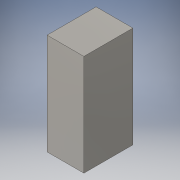
# Autodesk Inventor part: Motor
Saved by Autodesk Inventor 2016 (Build 200138000, 138)
## iProperties
Created: 2016-08-06
Part Number: Motor
Material: Stainless Steel
Document SubType Name: Modeling
Designer: Jorian Brusind
Density: 8 g/cm^3
Appearance: Semi-Polished
Author: Jorian Brusind
Autodesk Inventor part; units mm, degrees
ref_plane "YZ Plane" through (0, 0, 0) normal (1, 0, 0) x (0, 1, 0)
ref_plane "XZ Plane" through (0, 0, 0) normal (0, 1, 0) x (-1, 0, 0)
ref_plane "XY Plane" through (0, 0, 0) normal (0, 0, 1) x (1, 0, 0)
sketch "Sketch1" plane through (0, 0, 0) normal (0, 1, 0) x (-1, 0, 0)
  line L0 (0, 0) -> (-30.48, 0)
  line L1 (-30.48, 0) -> (-30.48, -40.64)
  line L2 (-30.48, -40.64) -> (0, -40.64)
  line L3 (0, -40.64) -> (0, 0)
  dimension "d3" = 30.48
  dimension "d4" = 40.64
  constraints: 8 end point, 2 parallel, 1 horizontal, 1 perpendicular
  measures "d3" distance of L2.end L1.end
  measures "d4" distance of L0.end L1.end
extrude "Extrusion2" add sketch "Sketch1" along normal blind 83.82
body "Solid2"
